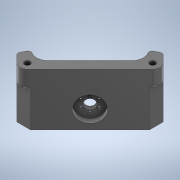
# Autodesk Inventor part: back_mount
Saved by Autodesk Inventor 2020 (Build 240168000, 168)
## iProperties
Created: 2023-12-16
Part Number: back_mount
Material: Пластик АБС
Document SubType Name: Modeling
Designer: denis
Density: 1.06 g/cm^3
Appearance: Гладкая — черная
Author: denis
Autodesk Inventor part; units mm, degrees
ref_plane "YZ Plane" through (0, 0, 0) normal (1, 0, 0) x (0, 1, 0)
ref_plane "XZ Plane" through (0, 0, 0) normal (0, 1, 0) x (-1, 0, 0)
ref_plane "XY Plane" through (0, 0, 0) normal (0, 0, 1) x (1, 0, 0)
sketch "Эскиз1" plane through (0, 0, 0) normal (0, 1, 0) x (-1, 0, 0)
  line L0 (34.2947, -76.014) -> (76.014, -34.2947)
  arc A0 (83.085, -34.2947) -> (76.014, -34.2947) centre (79.5495, -37.8302) ccw
  line L1 (83.085, -34.2947) -> (87.156, -38.3657)
  line L2 (46.3155, -73.8927) -> (73.8927, -46.3155)
  arc A1 (85.2064, -46.3155) -> (73.8927, -46.3155) centre (79.5495, -51.9723) ccw
  line L3 (85.2064, -46.3155) -> (87.5645, -48.6736)
  line L4 (92.5543, -49.5852) -> (94.5192, -45.7288)
  line L5 (87.156, -38.3657) -> (94.5192, -45.7288)
  line L6 (34.2947, -83.085) -> (38.3657, -87.156)
  arc A2 (34.2947, -76.014) -> (34.2947, -83.085) centre (37.8302, -79.5495) ccw
  arc A3 (46.3155, -73.8927) -> (46.3155, -85.2064) centre (51.9723, -79.5495) ccw
  line L7 (48.6736, -87.5645) -> (46.3155, -85.2064)
  line L8 (48.7014, -93.0224) -> (45.7288, -94.5192)
  line L9 (38.3657, -87.156) -> (45.7288, -94.5192)
  spline S0 degree 4 poles (87.5645, -48.6736) (88.1327, -49.2418) (88.8708, -49.8865) (89.7495, -50.471) (90.7127, -50.7263) (91.4939, -50.6999) (92.0261, -50.3682) (92.3519, -49.9478) (92.5543, -49.5852) knots 0 0 0 0 0 0.3763 0.501335 0.614666 0.722287 1 1 1 1 1
  spline S1 degree 4 poles (48.6736, -87.5645) (49.2196, -88.1111) (49.8318, -88.8375) (50.3553, -89.7359) (50.492, -90.7638) (50.3179, -91.6771) (49.7988, -92.3195) (49.2087, -92.7429) (48.7014, -93.0224) knots 0 0 0 0 0 0.349502 0.469309 0.582088 0.694155 1 1 1 1 1
  point P0 (0, 0)
  point P1 (49.5385, -88.5397)
  point P2 (50.0866, -89.3893)
  point P3 (50.374, -90.1304)
  point P4 (50.4468, -90.7861)
  point P5 (50.3313, -91.3833)
  point P6 (50.0252, -91.9468)
  point P7 (49.4982, -92.4922)
  point P8 (88.5759, -49.5937)
  point P9 (89.4338, -50.2024)
  point P10 (90.1559, -50.5529)
  point P11 (90.7644, -50.6948)
  point P12 (91.2858, -50.6665)
  point P13 (91.7467, -50.4838)
  point P14 (92.1672, -50.1352)
  constraints: 20 end point, 8 point on circle, 4 centre point, 1 coincident, 18 other
extrude "Выдавливание1" add sketch "Эскиз1" along normal blind 35
sketch "Эскиз2" plane through (-73.8927, 0, -46.3155) normal (-0.7071068, 0, -0.7071068) x (-0.7071068, 0, 0.7071068)
  line L0 (-39, 0) -> (0, 0) construction
  line L1 (0, 0) -> (0, 35) construction
  line L2 (-39, 35) -> (0, 35) construction
  line L3 (-39, 0) -> (-39, 35) construction
  line L4 (-39, 35) -> (0, 0) construction
  line L5 (0, 0) -> (0, 35) construction
  line L6 (0, 35) -> (-39, 0) construction
  circle A0 centre (-19.5, 17.5) radius 10.3
  circle A1 centre (-19.5, 17.5) radius 7.5 construction
  line L7 (-19.5, 0) -> (-19.5, 35) construction
  circle A2 centre (-19.5, 25) radius 1.25
  circle A3 centre (-25.9952, 21.25) radius 1.25
  circle A4 centre (-25.9952, 13.75) radius 1.25
  circle A5 centre (-19.5, 10) radius 1.25
  circle A6 centre (-13.0048, 13.75) radius 1.25
  circle A7 centre (-13.0048, 21.25) radius 1.25
  circle A8 centre (-19.5, 17.5) radius 5.5
  dimension "d3" = 15
  dimension "d2" = 20.6
  dimension "d4" = 2.5
  dimension "d7" = 360
  dimension "d9" = 11
  constraints: 8 centre point, 6 end point, 2 coincident, 2 midpoint, 1 point on line, 1 vertical alignment, 15 other
  measures "d2" diameter of A0
  measures "d4" diameter of A2
  measures "d9" diameter of A8
sketch "Эскиз3" plane through (0, 35, 0) normal (0, 1, 0) x (1, 0, 0)
  arc A0 (-83.085, 34.2947) -> (-76.014, 34.2947) centre (-79.5495, 37.8302) ccw construction
  arc A1 (-34.2947, 76.014) -> (-34.2947, 83.085) centre (-37.8302, 79.5495) ccw construction
  circle A2 centre (-79.5495, 37.8302) radius 1.9
  circle A3 centre (-37.8302, 79.5495) radius 1.9
  point P0 (0, 0)
  dimension "d17" = 3.8
  dimension "d18" = 3.8
  constraints: 2 centre point, 2 coincident
  measures "d17" diameter of A2
  measures "d18" diameter of A3
extrude "Выдавливание4" cut sketch "Эскиз3" against normal blind 40.5
sketch "Эскиз4" plane through (0, 0, 0) normal (0, -1, 0) x (1, 0, 0)
  arc A0 (-76.014, -34.2947) -> (-83.085, -34.2947) centre (-79.5495, -37.8302) ccw construction
  arc A1 (-34.2947, -83.085) -> (-34.2947, -76.014) centre (-37.8302, -79.5495) ccw construction
  circle A2 centre (-79.5495, -37.8302) radius 2
  circle A3 centre (-37.8302, -79.5495) radius 2
  point P0 (0, 0)
  dimension "d21" = 4
  dimension "d22" = 4
  constraints: 2 centre point, 2 coincident
  measures "d21" diameter of A2
  measures "d22" diameter of A3
extrude "Выдавливание5" cut sketch "Эскиз4" against normal blind 3.5
sketch "Эскиз5" plane through (-34.2947, 0, -76.014) normal (0.7071068, 0, 0.7071068) x (0.7071068, 0, -0.7071068)
  line L0 (-59, 0) -> (0, 0) construction
  line L1 (0, 0) -> (0, 35) construction
  line L2 (-59, 35) -> (0, 35) construction
  line L3 (-59, 0) -> (-59, 35) construction
  circle A0 centre (-29.5, 12) radius 3.25
  circle A1 centre (-29.5, 12) radius 5 construction
  circle A2 centre (-29.5, 12) radius 8.25
  circle A3 centre (-29.5, 17) radius 1.15
  line L4 (-29.5, 12) -> (-29.5, 35) construction
  circle A4 centre (-33.8301, 14.5) radius 1.15
  circle A5 centre (-33.8301, 9.5) radius 1.15
  circle A6 centre (-29.5, 7) radius 1.15
  circle A7 centre (-25.1699, 9.5) radius 1.15
  circle A8 centre (-25.1699, 14.5) radius 1.15
  point P0 (-29.5, 0)
  dimension "d30" = 10
  dimension "d29" = 6.5
  dimension "d31" = 16.5
  dimension "d32" = 2.3
  dimension "d35" = 360
  dimension "d44" = 12
  constraints: 8 centre point, 2 coincident, 2 end point, 1 midpoint, 1 point on line, 1 vertical, 1 vertical alignment, 15 other
  measures "d29" diameter of A0
  measures "d31" diameter of A2
  measures "d32" diameter of A3
  measures "d44" distance from line of L0 A0.centre
extrude "Выдавливание8" cut sketch "Эскиз5" against normal blind 13.5 contours A0 | A3 | A4 | A5 | A6 | A7 | A8
extrude "Выдавливание9" cut sketch "Эскиз5" against normal blind 4
chamfer "Фаска2" distance 0.5 angle 45 6 edges at (-60.9172, 17, -59.2909) (-63.9791, 14.5, -56.229) (-63.9791, 9.5, -56.229) (-60.9172, 7, -59.2909) (-57.8554, 9.5, -62.3528) (-57.8554, 14.5, -62.3528)
sketch "Эскиз6" plane through (-34.2947, 0, -76.014) normal (0.7071068, 0, 0.7071068) x (0.7071068, 0, -0.7071068)
  circle A0 centre (-29.5, 12) radius 8.25 construction
  point P0 (-29.5, 0)
sketch "Эскиз7" plane through (0, 35, 0) normal (0, 1, 0) x (1, 0, 0)
  circle A0 centre (0, 0) radius 97.5
  line L0 (-92.2037, 31.6976) -> (-101.2199, 49.6668)
  line L1 (-101.2199, 49.6668) -> (-45.4476, 101.4703)
  line L2 (-45.4476, 101.4703) -> (-33.8956, 91.4185)
  dimension "d45" = 195
  constraints: 6 end point, 2 point on circle, 1 centre point, 1 coincident
  measures "d45" diameter of A0
extrude "Выдавливание10" cut sketch "Эскиз7" against normal blind 40.5 contours A0 L0 L1 L2
fillet "Сопряжение1" radius 2 4 edges at (-46.6983, 17.5, -85.5892) (-40.0874, 17.5, -88.8777) (-85.5892, 17.5, -46.6983) (-88.8777, 17.5, -40.0874)
sketch "Эскиз8" plane through (0, 35, 0) normal (0, 1, 0) x (1, 0, 0)
  arc A0 (-88.2901, 41.3656) -> (-87.8932, 39.1028) centre (-86.479, 40.5171) ccw construction
  line L0 (-87.8932, 39.1028) -> (-83.085, 34.2947) construction
  arc A1 (-83.085, 34.2947) -> (-76.014, 34.2947) centre (-79.5495, 37.8302) ccw construction
  line L1 (-76.014, 34.2947) -> (-34.2947, 76.014) construction
  arc A2 (-34.2947, 76.014) -> (-34.2947, 83.085) centre (-37.8302, 79.5495) ccw construction
  line L2 (-34.2947, 83.085) -> (-39.1028, 87.8932) construction
  arc A3 (-39.1028, 87.8932) -> (-41.3656, 88.2901) centre (-40.5171, 86.479) ccw construction
  arc A4 (-41.3656, 88.2901) -> (-44.4874, 86.759) centre (0, 0) ccw construction
  arc A5 (-44.4874, 86.759) -> (-45.2544, 83.8933) centre (-43.5749, 84.9793) ccw construction
  arc A6 (-46.3155, 73.8927) -> (-45.2544, 83.8933) centre (-51.9723, 79.5495) ccw construction
  line L3 (-46.3155, 73.8927) -> (-73.8927, 46.3155) construction
  arc A7 (-83.8933, 45.2544) -> (-73.8927, 46.3155) centre (-79.5495, 51.9723) ccw construction
  arc A8 (-83.8933, 45.2544) -> (-86.759, 44.4874) centre (-84.9793, 43.5749) ccw construction
  arc A9 (-86.759, 44.4874) -> (-88.2901, 41.3656) centre (0, 0) ccw construction
  circle A10 centre (-37.8302, 79.5495) radius 1.9 construction
  circle A11 centre (-79.5495, 37.8302) radius 1.9 construction
  line L4 (-35.3302, 74.9784) -> (-35.3302, 84.1206)
  arc A12 (-34.2947, 76.014) -> (-34.2947, 83.085) centre (-37.8302, 79.5495) ccw construction
  line L5 (-76.014, 34.2947) -> (-34.2947, 76.014) construction
  line L6 (-46.3155, 73.8927) -> (-73.8927, 46.3155) construction
  line L7 (-60.1041, 60.1041) -> (-55.1543, 55.1543) construction
  line L8 (-49.3207, 60.988) -> (-60.988, 49.3207) construction
  line L9 (-35.3302, 74.9784) -> (-27.7018, 74.9784)
  line L10 (-27.7018, 74.9784) -> (-27.7018, 84.1206)
  line L11 (-27.7018, 84.1206) -> (-35.3302, 84.1206)
  line L12 (-35.3302, 84.1206) -> (-35.3302, 74.9784)
  line L13 (-74.9784, 35.3302) -> (-84.1206, 35.3302)
  line L14 (-74.9784, 35.3302) -> (-74.9784, 27.7018)
  line L15 (-74.9784, 27.7018) -> (-84.1206, 27.7018)
  line L16 (-84.1206, 27.7018) -> (-84.1206, 35.3302)
  point P0 (-32.8302, 79.5495)
  dimension "d49" = 2.5
  constraints: 20 end point, 5 symmetric about line, 2 midpoint, 2 parallel, 2 point on circle, 2 point on line, 1 horizontal, 1 perpendicular, 1 vertical
  measures "d49" distance from line of L4 point (-32.83, 79.55)
extrude "Выдавливание11" [suppressed]
sketch "Эскиз9" plane through (0, 0, 0) normal (0, -1, 0) x (1, 0, 0)
  line L0 (-74.9784, -35.3302) -> (-74.9784, -27.7018) projected
  line L1 (-74.9784, -35.3302) -> (-84.1206, -35.3302) projected
  line L2 (-84.1206, -27.7018) -> (-84.1206, -35.3302) projected
  line L3 (-74.9784, -27.7018) -> (-84.1206, -27.7018) projected
  line L4 (-27.7018, -74.9784) -> (-27.7018, -84.1206) projected
  line L5 (-27.7018, -84.1206) -> (-35.3302, -84.1206) projected
  line L6 (-35.3302, -74.9784) -> (-35.3302, -84.1206) projected
  line L7 (-35.3302, -74.9784) -> (-27.7018, -74.9784) projected
  point P0 (0, 0)
extrude "Выдавливание12" cut sketch "Эскиз9" against normal blind 23
chamfer "Фаска3" distance 2 angle 45 3 edges at (-32.8302, 23, -79.5495) (-34.8124, 23, -83.6028) (-34.8124, 23, -75.4962)
chamfer "Фаска4" distance 1.5 angle 45 3 edges at (-79.5495, 23, -32.8302) (-75.4962, 23, -34.8124) (-83.6028, 23, -34.8124)
